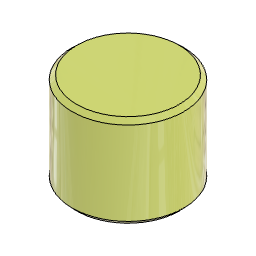
039426-02 MH Roller Cylinder (Autodesk Fusion 360 design; units mm, degrees)
Autodesk Fusion 360 part; units mm, degrees
sketch "Sketch1" plane through (0, 0, 0) normal (0, 0, 1) x (1, 0, 0)
  circle A0 centre (0, 0) radius 31.75
  dimension "d3" = 63.5
  constraint coincident A0.centre origin
  measures "d3" diameter of A0
extrude "Extrude1" add sketch "Sketch1" along normal blind 52.5018
chamfer "Chamfer1" distance 2.54 distance2 2.3622 2 edges at (-29.6014, -11.4813, 52.5018) (-29.6014, -11.4813, 0) measured on face at (-7.9711, 4.3562, 52.5018) measured on face at (31.5922, -3.1613, 17.5006)
equation "RollerDiameter = 2 1/2\""
equation "RollerWidth = 2.067 in"
equation "d3 = RollerDiameter"
equation "d4 = RollerWidth"
equation "RollerBevel = ( 1 / 8 ) * 1 in"
